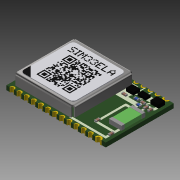
# Autodesk Inventor part: SIM28M
Saved by Autodesk Inventor 2015 SP1 (Build 190203100, 203)
## iProperties
Created: 2015-01-28
Part Number: SIM28M
Material: Типовые
Document SubType Name: Modeling
Designer: Danil
Density: 1 g/cm^3
Appearance: Default
Author: Danil
Autodesk Inventor part; units mm, degrees
(part 1 of 3)
ref_plane "YZ Plane" through (0, 0, 0) normal (1, 0, 0) x (0, 1, 0)
ref_plane "XZ Plane" through (0, 0, 0) normal (0, 1, 0) x (-1, 0, 0)
ref_plane "XY Plane" through (0, 0, 0) normal (0, 0, 1) x (1, 0, 0)
sketch "Эскиз4" plane through (0, 0, 0) normal (0, 0, 1) x (1, 0, 0)
  arc A0 (4.53, 4.775) -> (5.07, 4.775) centre (4.8, 4.775) ccw
  line L0 (5.07, 4.775) -> (5.1, 4.775)
  line L1 (5.1, 4.775) -> (5.1, 4.375) construction
  line L2 (5.1, 4.375) -> (4.5, 4.375) construction
  line L3 (4.5, 4.375) -> (4.5, 4.775) construction
  line L4 (4.5, 4.775) -> (4.53, 4.775)
  arc A1 (4.5, 4.675) -> (5.1, 4.675) centre (4.8, 4.675) ccw
  line L5 (4.8, 4.675) -> (5.1, 4.675) construction
  line L6 (4.8, 4.675) -> (4.5, 4.675) construction
  line L7 (4.5, 4.675) -> (4.5, 4.775)
  line L8 (5.1, 4.775) -> (5.1, 4.675)
  arc A2 (5.68, 4.775) -> (6.22, 4.775) centre (5.95, 4.775) ccw
  arc A3 (5.5, 4.775) -> (6.4, 4.775) centre (5.95, 4.775) ccw
  line L9 (5.5, 4.775) -> (5.68, 4.775)
  line L10 (6.22, 4.775) -> (6.4, 4.775)
  line L11 (-6.975, -4.775) -> (6.975, -4.775)
  line L12 (6.975, -4.775) -> (6.975, 4.775)
  line L13 (6.975, 4.775) -> (-6.975, 4.775)
  line L14 (-6.975, 4.775) -> (-6.975, -4.775)
  line L15 (-6.975, -4.775) -> (6.975, 4.775) construction
  line L16 (6.975, -4.775) -> (-6.975, 4.775) construction
  line L17 (4.53, 4.775) -> (5.07, 4.775)
  line L18 (5.68, 4.775) -> (6.22, 4.775)
  line L19 (0, 0) -> (6.975, 0) construction
  arc A4 (3.53, 4.775) -> (4.07, 4.775) centre (3.8, 4.775) ccw
  line L20 (4.07, 4.775) -> (4.1, 4.775)
  line L21 (4.1, 4.775) -> (4.1, 4.375) construction
  line L22 (4.1, 4.375) -> (3.5, 4.375) construction
  line L23 (3.5, 4.375) -> (3.5, 4.775) construction
  line L24 (3.5, 4.775) -> (3.53, 4.775)
  arc A5 (3.5, 4.675) -> (4.1, 4.675) centre (3.8, 4.675) ccw
  line L25 (3.8, 4.675) -> (4.1, 4.675) construction
  line L26 (3.8, 4.675) -> (3.5, 4.675) construction
  line L27 (3.5, 4.675) -> (3.5, 4.775)
  line L28 (4.1, 4.775) -> (4.1, 4.675)
  line L29 (3.53, 4.775) -> (4.07, 4.775)
  line L30 (2.5, 4.775) -> (2.53, 4.775)
  line L31 (2.8, 4.675) -> (2.5, 4.675) construction
  line L32 (2.53, 4.775) -> (3.07, 4.775)
  arc A6 (2.53, 4.775) -> (3.07, 4.775) centre (2.8, 4.775) ccw
  line L33 (3.07, 4.775) -> (3.1, 4.775)
  line L34 (3.1, 4.775) -> (3.1, 4.375) construction
  line L35 (3.1, 4.375) -> (2.5, 4.375) construction
  line L36 (2.8, 4.675) -> (3.1, 4.675) construction
  arc A7 (2.5, 4.675) -> (3.1, 4.675) centre (2.8, 4.675) ccw
  line L37 (2.5, 4.375) -> (2.5, 4.775) construction
  line L38 (2.5, 4.675) -> (2.5, 4.775)
  line L39 (3.1, 4.775) -> (3.1, 4.675)
  line L40 (1.5, 4.775) -> (1.53, 4.775)
  line L41 (1.8, 4.675) -> (1.5, 4.675) construction
  line L42 (1.53, 4.775) -> (2.07, 4.775)
  arc A8 (1.53, 4.775) -> (2.07, 4.775) centre (1.8, 4.775) ccw
  line L43 (2.07, 4.775) -> (2.1, 4.775)
  line L44 (2.1, 4.775) -> (2.1, 4.375) construction
  line L45 (2.1, 4.375) -> (1.5, 4.375) construction
  line L46 (1.8, 4.675) -> (2.1, 4.675) construction
  arc A9 (1.5, 4.675) -> (2.1, 4.675) centre (1.8, 4.675) ccw
  line L47 (1.5, 4.375) -> (1.5, 4.775) construction
  line L48 (1.5, 4.675) -> (1.5, 4.775)
  line L49 (2.1, 4.775) -> (2.1, 4.675)
  line L50 (0.5, 4.775) -> (0.53, 4.775)
  line L51 (0.8, 4.675) -> (0.5, 4.675) construction
  line L52 (0.53, 4.775) -> (1.07, 4.775)
  arc A10 (0.53, 4.775) -> (1.07, 4.775) centre (0.8, 4.775) ccw
  line L53 (1.07, 4.775) -> (1.1, 4.775)
  line L54 (1.1, 4.775) -> (1.1, 4.375) construction
  line L55 (1.1, 4.375) -> (0.5, 4.375) construction
  line L56 (0.8, 4.675) -> (1.1, 4.675) construction
  arc A11 (0.5, 4.675) -> (1.1, 4.675) centre (0.8, 4.675) ccw
  line L57 (0.5, 4.375) -> (0.5, 4.775) construction
  line L58 (0.5, 4.675) -> (0.5, 4.775)
  line L59 (1.1, 4.775) -> (1.1, 4.675)
  line L60 (-0.5, 4.775) -> (-0.47, 4.775)
  line L61 (-0.2, 4.675) -> (-0.5, 4.675) construction
  line L62 (-0.47, 4.775) -> (0.07, 4.775)
  arc A12 (-0.47, 4.775) -> (0.07, 4.775) centre (-0.2, 4.775) ccw
  line L63 (0.07, 4.775) -> (0.1, 4.775)
  line L64 (0.1, 4.775) -> (0.1, 4.375) construction
  line L65 (0.1, 4.375) -> (-0.5, 4.375) construction
  line L66 (-0.2, 4.675) -> (0.1, 4.675) construction
  arc A13 (-0.5, 4.675) -> (0.1, 4.675) centre (-0.2, 4.675) ccw
  line L67 (-0.5, 4.375) -> (-0.5, 4.775) construction
  line L68 (-0.5, 4.675) -> (-0.5, 4.775)
  line L69 (0.1, 4.775) -> (0.1, 4.675)
  line L70 (-1.5, 4.775) -> (-1.47, 4.775)
  line L71 (-1.2, 4.675) -> (-1.5, 4.675) construction
  line L72 (-1.47, 4.775) -> (-0.93, 4.775)
  arc A14 (-1.47, 4.775) -> (-0.93, 4.775) centre (-1.2, 4.775) ccw
  line L73 (-0.93, 4.775) -> (-0.9, 4.775)
  line L74 (-0.9, 4.775) -> (-0.9, 4.375) construction
  line L75 (-0.9, 4.375) -> (-1.5, 4.375) construction
  line L76 (-1.2, 4.675) -> (-0.9, 4.675) construction
  arc A15 (-1.5, 4.675) -> (-0.9, 4.675) centre (-1.2, 4.675) ccw
  line L77 (-1.5, 4.375) -> (-1.5, 4.775) construction
  line L78 (-1.5, 4.675) -> (-1.5, 4.775)
  line L79 (-0.9, 4.775) -> (-0.9, 4.675)
  line L80 (-2.5, 4.775) -> (-2.47, 4.775)
  line L81 (-2.2, 4.675) -> (-2.5, 4.675) construction
  line L82 (-2.47, 4.775) -> (-1.93, 4.775)
  arc A16 (-2.47, 4.775) -> (-1.93, 4.775) centre (-2.2, 4.775) ccw
  line L83 (-1.93, 4.775) -> (-1.9, 4.775)
  line L84 (-1.9, 4.775) -> (-1.9, 4.375) construction
  line L85 (-1.9, 4.375) -> (-2.5, 4.375) construction
  line L86 (-2.2, 4.675) -> (-1.9, 4.675) construction
  arc A17 (-2.5, 4.675) -> (-1.9, 4.675) centre (-2.2, 4.675) ccw
  line L87 (-2.5, 4.375) -> (-2.5, 4.775) construction
  line L88 (-2.5, 4.675) -> (-2.5, 4.775)
  line L89 (-1.9, 4.775) -> (-1.9, 4.675)
  line L90 (-3.5, 4.775) -> (-3.47, 4.775)
  line L91 (-3.2, 4.675) -> (-3.5, 4.675) construction
  line L92 (-3.47, 4.775) -> (-2.93, 4.775)
  arc A18 (-3.47, 4.775) -> (-2.93, 4.775) centre (-3.2, 4.775) ccw
  line L93 (-2.93, 4.775) -> (-2.9, 4.775)
  line L94 (-2.9, 4.775) -> (-2.9, 4.375) construction
  line L95 (-2.9, 4.375) -> (-3.5, 4.375) construction
  line L96 (-3.2, 4.675) -> (-2.9, 4.675) construction
  arc A19 (-3.5, 4.675) -> (-2.9, 4.675) centre (-3.2, 4.675) ccw
  line L97 (-3.5, 4.375) -> (-3.5, 4.775) construction
  line L98 (-3.5, 4.675) -> (-3.5, 4.775)
  line L99 (-2.9, 4.775) -> (-2.9, 4.675)
  line L100 (-4.5, 4.775) -> (-4.47, 4.775)
  line L101 (-4.2, 4.675) -> (-4.5, 4.675) construction
  line L102 (-4.47, 4.775) -> (-3.93, 4.775)
  arc A20 (-4.47, 4.775) -> (-3.93, 4.775) centre (-4.2, 4.775) ccw
  line L103 (-3.93, 4.775) -> (-3.9, 4.775)
  line L104 (-3.9, 4.775) -> (-3.9, 4.375) construction
  line L105 (-3.9, 4.375) -> (-4.5, 4.375) construction
  line L106 (-4.2, 4.675) -> (-3.9, 4.675) construction
  arc A21 (-4.5, 4.675) -> (-3.9, 4.675) centre (-4.2, 4.675) ccw
  line L107 (-4.5, 4.375) -> (-4.5, 4.775) construction
  line L108 (-4.5, 4.675) -> (-4.5, 4.775)
  line L109 (-3.9, 4.775) -> (-3.9, 4.675)
  line L110 (-5.5, 4.775) -> (-5.47, 4.775)
  line L111 (-5.2, 4.675) -> (-5.5, 4.675) construction
  line L112 (-5.47, 4.775) -> (-4.93, 4.775)
  arc A22 (-5.47, 4.775) -> (-4.93, 4.775) centre (-5.2, 4.775) ccw
  line L113 (-4.93, 4.775) -> (-4.9, 4.775)
  line L114 (-4.9, 4.775) -> (-4.9, 4.375) construction
  line L115 (-4.9, 4.375) -> (-5.5, 4.375) construction
  line L116 (-5.2, 4.675) -> (-4.9, 4.675) construction
  arc A23 (-5.5, 4.675) -> (-4.9, 4.675) centre (-5.2, 4.675) ccw
  line L117 (-5.5, 4.375) -> (-5.5, 4.775) construction
  line L118 (-5.5, 4.675) -> (-5.5, 4.775)
  line L119 (-4.9, 4.775) -> (-4.9, 4.675)
  line L120 (-6.5, 4.775) -> (-6.47, 4.775)
  line L121 (-6.2, 4.675) -> (-6.5, 4.675) construction
  line L122 (-6.47, 4.775) -> (-5.93, 4.775)
  arc A24 (-6.47, 4.775) -> (-5.93, 4.775) centre (-6.2, 4.775) ccw
  line L123 (-5.93, 4.775) -> (-5.9, 4.775)
  line L124 (-5.9, 4.775) -> (-5.9, 4.375) construction
  line L125 (-5.9, 4.375) -> (-6.5, 4.375) construction
  line L126 (-6.2, 4.675) -> (-5.9, 4.675) construction
  arc A25 (-6.5, 4.675) -> (-5.9, 4.675) centre (-6.2, 4.675) ccw
  line L127 (-6.5, 4.375) -> (-6.5, 4.775) construction
  line L128 (-6.5, 4.675) -> (-6.5, 4.775)
  line L129 (-5.9, 4.775) -> (-5.9, 4.675)
  line L130 (-6.875, 1.7) -> (-6.975, 1.7)
  line L131 (-6.575, 1.7) -> (-6.975, 1.7) construction
  line L132 (-6.975, 1.7) -> (-6.975, 1.73)
  line L133 (-6.975, 2.27) -> (-6.975, 2.3)
  arc A26 (-6.875, 1.7) -> (-6.875, 2.3) centre (-6.875, 2) ccw
  line L134 (-6.875, 2) -> (-6.875, 2.3) construction
  line L135 (-6.975, 2.3) -> (-6.875, 2.3)
  line L136 (-6.975, 2.3) -> (-6.575, 2.3) construction
  line L137 (-6.875, 2) -> (-6.875, 1.7) construction
  line L138 (-6.975, 1.73) -> (-6.975, 2.27)
  arc A27 (-6.975, 1.73) -> (-6.975, 2.27) centre (-6.975, 2) ccw
  line L139 (-6.575, 2.3) -> (-6.575, 1.7) construction
  line L140 (-6.975, 1.27) -> (-6.975, 1.3)
  line L141 (-6.875, 1) -> (-6.875, 1.3) construction
  line L142 (-6.975, 1.3) -> (-6.875, 1.3)
  line L143 (-6.975, 1.3) -> (-6.575, 1.3) construction
  line L144 (-6.975, 0.73) -> (-6.975, 1.27)
  arc A28 (-6.975, 0.73) -> (-6.975, 1.27) centre (-6.975, 1) ccw
  line L145 (-6.575, 1.3) -> (-6.575, 0.7) construction
  arc A29 (-6.875, 0.7) -> (-6.875, 1.3) centre (-6.875, 1) ccw
  line L146 (-6.875, 1) -> (-6.875, 0.7) construction
  line L147 (-6.975, 0.7) -> (-6.975, 0.73)
  line L148 (-6.875, 0.7) -> (-6.975, 0.7)
  line L149 (-6.575, 0.7) -> (-6.975, 0.7) construction
  line L150 (-6.975, 0.27) -> (-6.975, 0.3)
  line L151 (-6.875, 0) -> (-6.875, 0.3) construction
  line L152 (-6.975, 0.3) -> (-6.875, 0.3)
  line L153 (-6.975, 0.3) -> (-6.575, 0.3) construction
  line L154 (-6.975, -0.27) -> (-6.975, 0.27)
  arc A30 (-6.975, -0.27) -> (-6.975, 0.27) centre (-6.975, 0) ccw
  line L155 (-6.575, 0.3) -> (-6.575, -0.3) construction
  arc A31 (-6.875, -0.3) -> (-6.875, 0.3) centre (-6.875, 0) ccw
  line L156 (-6.875, 0) -> (-6.875, -0.3) construction
  line L157 (-6.975, -0.3) -> (-6.975, -0.27)
  line L158 (-6.875, -0.3) -> (-6.975, -0.3)
  line L159 (-6.575, -0.3) -> (-6.975, -0.3) construction
  line L160 (-6.975, -0.73) -> (-6.975, -0.7)
  line L161 (-6.875, -1) -> (-6.875, -0.7) construction
  line L162 (-6.975, -0.7) -> (-6.875, -0.7)
  line L163 (-6.975, -0.7) -> (-6.575, -0.7) construction
  line L164 (-6.975, -1.27) -> (-6.975, -0.73)
  arc A32 (-6.975, -1.27) -> (-6.975, -0.73) centre (-6.975, -1) ccw
  line L165 (-6.575, -0.7) -> (-6.575, -1.3) construction
  arc A33 (-6.875, -1.3) -> (-6.875, -0.7) centre (-6.875, -1) ccw
  line L166 (-6.875, -1) -> (-6.875, -1.3) construction
  line L167 (-6.975, -1.3) -> (-6.975, -1.27)
  line L168 (-6.875, -1.3) -> (-6.975, -1.3)
  line L169 (-6.575, -1.3) -> (-6.975, -1.3) construction
  line L170 (-6.975, -1.73) -> (-6.975, -1.7)
  line L171 (-6.875, -2) -> (-6.875, -1.7) construction
  line L172 (-6.975, -1.7) -> (-6.875, -1.7)
  line L173 (-6.975, -1.7) -> (-6.575, -1.7) construction
  line L174 (-6.975, -2.27) -> (-6.975, -1.73)
  arc A34 (-6.975, -2.27) -> (-6.975, -1.73) centre (-6.975, -2) ccw
  line L175 (-6.575, -1.7) -> (-6.575, -2.3) construction
  arc A35 (-6.875, -2.3) -> (-6.875, -1.7) centre (-6.875, -2) ccw
  line L176 (-6.875, -2) -> (-6.875, -2.3) construction
  line L177 (-6.975, -2.3) -> (-6.975, -2.27)
  line L178 (-6.875, -2.3) -> (-6.975, -2.3)
  line L179 (-6.575, -2.3) -> (-6.975, -2.3) construction
  arc A36 (5.07, -4.775) -> (4.53, -4.775) centre (4.8, -4.775) ccw
  line L180 (5.07, -4.775) -> (5.1, -4.775)
  line L181 (5.1, -4.775) -> (5.1, -4.375) construction
  line L182 (5.1, -4.375) -> (4.5, -4.375) construction
  line L183 (4.5, -4.375) -> (4.5, -4.775) construction
  line L184 (4.5, -4.775) -> (4.53, -4.775)
  arc A37 (5.1, -4.675) -> (4.5, -4.675) centre (4.8, -4.675) ccw
  line L185 (4.8, -4.675) -> (5.1, -4.675) construction
  line L186 (4.8, -4.675) -> (4.5, -4.675) construction
  line L187 (4.5, -4.675) -> (4.5, -4.775)
  line L188 (5.1, -4.775) -> (5.1, -4.675)
  arc A38 (6.22, -4.775) -> (5.68, -4.775) centre (5.95, -4.775) ccw
  arc A39 (6.4, -4.775) -> (5.5, -4.775) centre (5.95, -4.775) ccw
  line L189 (5.5, -4.775) -> (5.68, -4.775)
  line L190 (6.22, -4.775) -> (6.4, -4.775)
  line L191 (4.53, -4.775) -> (5.07, -4.775)
  line L192 (5.68, -4.775) -> (6.22, -4.775)
  line L193 (3.5, -4.775) -> (3.53, -4.775)
  line L194 (3.8, -4.675) -> (3.5, -4.675) construction
  line L195 (3.53, -4.775) -> (4.07, -4.775)
  arc A40 (4.07, -4.775) -> (3.53, -4.775) centre (3.8, -4.775) ccw
  line L196 (4.07, -4.775) -> (4.1, -4.775)
  line L197 (4.1, -4.775) -> (4.1, -4.375) construction
  line L198 (4.1, -4.375) -> (3.5, -4.375) construction
  line L199 (3.8, -4.675) -> (4.1, -4.675) construction
  arc A41 (4.1, -4.675) -> (3.5, -4.675) centre (3.8, -4.675) ccw
  line L200 (3.5, -4.375) -> (3.5, -4.775) construction
  line L201 (3.5, -4.675) -> (3.5, -4.775)
  line L202 (4.1, -4.775) -> (4.1, -4.675)
  line L203 (2.5, -4.675) -> (2.5, -4.775)
  line L204 (2.5, -4.375) -> (2.5, -4.775) construction
  line L205 (2.5, -4.775) -> (2.53, -4.775)
  line L206 (3.07, -4.775) -> (3.1, -4.775)
  arc A42 (3.1, -4.675) -> (2.5, -4.675) centre (2.8, -4.675) ccw
  line L207 (2.8, -4.675) -> (3.1, -4.675) construction
  line L208 (3.1, -4.775) -> (3.1, -4.675)
  line L209 (3.1, -4.775) -> (3.1, -4.375) construction
  line L210 (2.8, -4.675) -> (2.5, -4.675) construction
  line L211 (2.53, -4.775) -> (3.07, -4.775)
  arc A43 (3.07, -4.775) -> (2.53, -4.775) centre (2.8, -4.775) ccw
  line L212 (3.1, -4.375) -> (2.5, -4.375) construction
  line L213 (1.5, -4.675) -> (1.5, -4.775)
  line L214 (1.5, -4.375) -> (1.5, -4.775) construction
  line L215 (1.5, -4.775) -> (1.53, -4.775)
  line L216 (2.07, -4.775) -> (2.1, -4.775)
  arc A44 (2.1, -4.675) -> (1.5, -4.675) centre (1.8, -4.675) ccw
  line L217 (1.8, -4.675) -> (2.1, -4.675) construction
  line L218 (2.1, -4.775) -> (2.1, -4.675)
  line L219 (2.1, -4.775) -> (2.1, -4.375) construction
  line L220 (1.8, -4.675) -> (1.5, -4.675) construction
  line L221 (1.53, -4.775) -> (2.07, -4.775)
  arc A45 (2.07, -4.775) -> (1.53, -4.775) centre (1.8, -4.775) ccw
  line L222 (2.1, -4.375) -> (1.5, -4.375) construction
  line L223 (0.5, -4.675) -> (0.5, -4.775)
  line L224 (0.5, -4.375) -> (0.5, -4.775) construction
  line L225 (0.5, -4.775) -> (0.53, -4.775)
  line L226 (1.07, -4.775) -> (1.1, -4.775)
  arc A46 (1.1, -4.675) -> (0.5, -4.675) centre (0.8, -4.675) ccw
  line L227 (0.8, -4.675) -> (1.1, -4.675) construction
  line L228 (1.1, -4.775) -> (1.1, -4.675)
  line L229 (1.1, -4.775) -> (1.1, -4.375) construction
  line L230 (0.8, -4.675) -> (0.5, -4.675) construction
  line L231 (0.53, -4.775) -> (1.07, -4.775)
  arc A47 (1.07, -4.775) -> (0.53, -4.775) centre (0.8, -4.775) ccw
  line L232 (1.1, -4.375) -> (0.5, -4.375) construction
  line L233 (-0.5, -4.675) -> (-0.5, -4.775)
  line L234 (-0.5, -4.375) -> (-0.5, -4.775) construction
  line L235 (-0.5, -4.775) -> (-0.47, -4.775)
  line L236 (0.07, -4.775) -> (0.1, -4.775)
  arc A48 (0.1, -4.675) -> (-0.5, -4.675) centre (-0.2, -4.675) ccw
  line L237 (-0.2, -4.675) -> (0.1, -4.675) construction
  line L238 (0.1, -4.775) -> (0.1, -4.675)
  line L239 (0.1, -4.775) -> (0.1, -4.375) construction
  line L240 (-0.2, -4.675) -> (-0.5, -4.675) construction
  line L241 (-0.47, -4.775) -> (0.07, -4.775)
  arc A49 (0.07, -4.775) -> (-0.47, -4.775) centre (-0.2, -4.775) ccw
  line L242 (0.1, -4.375) -> (-0.5, -4.375) construction
  line L243 (-1.5, -4.675) -> (-1.5, -4.775)
  line L244 (-1.5, -4.375) -> (-1.5, -4.775) construction
  line L245 (-1.5, -4.775) -> (-1.47, -4.775)
  line L246 (-0.93, -4.775) -> (-0.9, -4.775)
  arc A50 (-0.9, -4.675) -> (-1.5, -4.675) centre (-1.2, -4.675) ccw
  line L247 (-1.2, -4.675) -> (-0.9, -4.675) construction
  line L248 (-0.9, -4.775) -> (-0.9, -4.675)
  line L249 (-0.9, -4.775) -> (-0.9, -4.375) construction
  line L250 (-1.2, -4.675) -> (-1.5, -4.675) construction
  line L251 (-1.47, -4.775) -> (-0.93, -4.775)
  arc A51 (-0.93, -4.775) -> (-1.47, -4.775) centre (-1.2, -4.775) ccw
  line L252 (-0.9, -4.375) -> (-1.5, -4.375) construction
  line L253 (-2.5, -4.675) -> (-2.5, -4.775)
  line L254 (-2.5, -4.375) -> (-2.5, -4.775) construction
  line L255 (-2.5, -4.775) -> (-2.47, -4.775)
  line L256 (-1.93, -4.775) -> (-1.9, -4.775)
  arc A52 (-1.9, -4.675) -> (-2.5, -4.675) centre (-2.2, -4.675) ccw
  line L257 (-2.2, -4.675) -> (-1.9, -4.675) construction
  line L258 (-1.9, -4.775) -> (-1.9, -4.675)
  line L259 (-1.9, -4.775) -> (-1.9, -4.375) construction
  line L260 (-2.2, -4.675) -> (-2.5, -4.675) construction
  line L261 (-2.47, -4.775) -> (-1.93, -4.775)
  arc A53 (-1.93, -4.775) -> (-2.47, -4.775) centre (-2.2, -4.775) ccw
  line L262 (-1.9, -4.375) -> (-2.5, -4.375) construction
  line L263 (-3.5, -4.675) -> (-3.5, -4.775)
  line L264 (-3.5, -4.375) -> (-3.5, -4.775) construction
  line L265 (-3.5, -4.775) -> (-3.47, -4.775)
  line L266 (-2.93, -4.775) -> (-2.9, -4.775)
  arc A54 (-2.9, -4.675) -> (-3.5, -4.675) centre (-3.2, -4.675) ccw
  line L267 (-3.2, -4.675) -> (-2.9, -4.675) construction
  line L268 (-2.9, -4.775) -> (-2.9, -4.675)
  line L269 (-2.9, -4.775) -> (-2.9, -4.375) construction
  line L270 (-3.2, -4.675) -> (-3.5, -4.675) construction
  line L271 (-3.47, -4.775) -> (-2.93, -4.775)
  arc A55 (-2.93, -4.775) -> (-3.47, -4.775) centre (-3.2, -4.775) ccw
  line L272 (-2.9, -4.375) -> (-3.5, -4.375) construction
  line L273 (-4.5, -4.675) -> (-4.5, -4.775)
  line L274 (-4.5, -4.375) -> (-4.5, -4.775) construction
  line L275 (-4.5, -4.775) -> (-4.47, -4.775)
  line L276 (-3.93, -4.775) -> (-3.9, -4.775)
  arc A56 (-3.9, -4.675) -> (-4.5, -4.675) centre (-4.2, -4.675) ccw
  line L277 (-4.2, -4.675) -> (-3.9, -4.675) construction
  line L278 (-3.9, -4.775) -> (-3.9, -4.675)
  line L279 (-3.9, -4.775) -> (-3.9, -4.375) construction
  line L280 (-4.2, -4.675) -> (-4.5, -4.675) construction
  line L281 (-4.47, -4.775) -> (-3.93, -4.775)
  arc A57 (-3.93, -4.775) -> (-4.47, -4.775) centre (-4.2, -4.775) ccw
  line L282 (-3.9, -4.375) -> (-4.5, -4.375) construction
  line L283 (-5.5, -4.675) -> (-5.5, -4.775)
  line L284 (-5.5, -4.375) -> (-5.5, -4.775) construction
  line L285 (-5.5, -4.775) -> (-5.47, -4.775)
  line L286 (-4.93, -4.775) -> (-4.9, -4.775)
  arc A58 (-4.9, -4.675) -> (-5.5, -4.675) centre (-5.2, -4.675) ccw
  line L287 (-5.2, -4.675) -> (-4.9, -4.675) construction
  line L288 (-4.9, -4.775) -> (-4.9, -4.675)
  line L289 (-4.9, -4.775) -> (-4.9, -4.375) construction
  line L290 (-5.2, -4.675) -> (-5.5, -4.675) construction
  line L291 (-5.47, -4.775) -> (-4.93, -4.775)
  arc A59 (-4.93, -4.775) -> (-5.47, -4.775) centre (-5.2, -4.775) ccw
  line L292 (-4.9, -4.375) -> (-5.5, -4.375) construction
  line L293 (-6.5, -4.675) -> (-6.5, -4.775)
  line L294 (-6.5, -4.375) -> (-6.5, -4.775) construction
  line L295 (-6.5, -4.775) -> (-6.47, -4.775)
  line L296 (-5.93, -4.775) -> (-5.9, -4.775)
  arc A60 (-5.9, -4.675) -> (-6.5, -4.675) centre (-6.2, -4.675) ccw
  line L297 (-6.2, -4.675) -> (-5.9, -4.675) construction
  line L298 (-5.9, -4.775) -> (-5.9, -4.675)
  line L299 (-5.9, -4.775) -> (-5.9, -4.375) construction
  line L300 (-6.2, -4.675) -> (-6.5, -4.675) construction
  line L301 (-6.47, -4.775) -> (-5.93, -4.775)
  arc A61 (-5.93, -4.775) -> (-6.47, -4.775) centre (-6.2, -4.775) ccw
  line L302 (-5.9, -4.375) -> (-6.5, -4.375) construction
  point P0 (4.8, 4.375)
  point P1 (3.8, 4.375)
  point P2 (2.8, 4.375)
  point P3 (1.8, 4.375)
  point P4 (0.8, 4.375)
  point P5 (-0.2, 4.375)
  point P6 (-1.2, 4.375)
  point P7 (-2.2, 4.375)
  point P8 (-3.2, 4.375)
  point P9 (-4.2, 4.375)
  point P10 (-5.2, 4.375)
  point P11 (-6.2, 4.375)
  point P12 (-6.575, 2)
  point P13 (-6.575, 1)
  point P14 (-6.575, 0)
  point P15 (-6.575, -1)
  point P16 (-6.575, -2)
  point P17 (-6.975, 0)
  point P18 (4.8, -4.375)
  point P19 (3.8, -4.375)
  point P20 (2.8, -4.375)
  point P21 (1.8, -4.375)
  point P22 (0.8, -4.375)
  point P23 (-0.2, -4.375)
  point P24 (-1.2, -4.375)
  point P25 (-2.2, -4.375)
  point P26 (-3.2, -4.375)
  point P27 (-4.2, -4.375)
  point P28 (-5.2, -4.375)
  point P29 (-6.2, -4.375)
  dimension "d738" = 0.27
  dimension "d741" = 0.6
  dimension "d742" = 0.4
  dimension "d809" = 0.27
  dimension "d826" = 0.45
  dimension "d830" = 1.15
  dimension "d872" = 13.95
  dimension "d873" = 9.55
  dimension "d874" = 0.27
  dimension "d875" = 0.6
  dimension "d876" = 0.4
  dimension "d877" = 1
  dimension "d878" = 0.27
  dimension "d879" = 0.6
  dimension "d880" = 0.4
  dimension "d881" = 0.27
  dimension "d882" = 0.6
  dimension "d883" = 0.4
  dimension "d884" = 0.27
  dimension "d885" = 0.6
  dimension "d886" = 0.4
  dimension "d887" = 0.27
  dimension "d888" = 0.6
  dimension "d889" = 0.4
  dimension "d890" = 0.27
  dimension "d891" = 0.6
  dimension "d892" = 0.4
  dimension "d893" = 0.27
  dimension "d894" = 0.6
  dimension "d895" = 0.4
  dimension "d896" = 0.27
  dimension "d897" = 0.6
  dimension "d898" = 0.4
  dimension "d899" = 0.27
  dimension "d900" = 0.6
  dimension "d901" = 0.4
  dimension "d902" = 0.27
  dimension "d903" = 0.6
  dimension "d904" = 0.4
  dimension "d905" = 0.27
  dimension "d906" = 0.6
  dimension "d907" = 0.4
  dimension "d908" = 1
  dimension "d909" = 0.775
  dimension "d910" = 1
  dimension "d911" = 1
  dimension "d912" = 1
  dimension "d913" = 1
  dimension "d914" = 1
  dimension "d915" = 1
  dimension "d916" = 1
  dimension "d917" = 1
  dimension "d918" = 1
  dimension "d919" = 0.27
  dimension "d920" = 0.6
  dimension "d921" = 0.4
  dimension "d923" = 2.775
  dimension "d924" = 0.27
  dimension "d925" = 0.6
  dimension "d926" = 0.4
  dimension "d927" = 0.27
  dimension "d928" = 0.6
  dimension "d929" = 0.4
  dimension "d930" = 0.27
  constraints: 604 end point, 149 symmetric about line, 141 point on circle, 91 point on line, 86 perpendicular, 62 centre point, 57 horizontal alignment, 39 midpoint, 35 parallel, 18 collinear, 17 horizontal, 17 vertical alignment, 7 coincident, 43 other
  measures "d738" radius of A0
  measures "d741" distance between parallel lines of L1 L3
  measures "d742" distance of L2.end L3.end
  measures "d809" radius of A2
  measures "d826" radius of A3
  measures "d830" distance of A0.centre A2.centre
  measures "d872" distance of L14.start L12.end
  measures "d873" distance of L12.end L11.end
  measures "d874" radius of A4
  measures "d875" distance between parallel lines of L21 L23
  measures "d876" distance of L22.end L24.start
  measures "d877" distance of A0.centre A4.centre
  measures "d878" radius of A6
  measures "d879" distance between parallel lines of L34 L37
  measures "d880" distance of L37.start L38.end
  measures "d881" radius of A8
  measures "d882" distance between parallel lines of L44 L47
  measures "d883" distance of L47.start L48.end
  measures "d884" radius of A10
  measures "d885" distance between parallel lines of L54 L57
  measures "d886" distance of L57.start L58.end
  measures "d887" radius of A12
  measures "d888" distance between parallel lines of L64 L67
  measures "d889" distance of L67.start L68.end
  measures "d890" radius of A14
  measures "d891" distance between parallel lines of L74 L77
  measures "d892" distance of L77.start L78.end
  measures "d893" radius of A16
  measures "d894" distance between parallel lines of L84 L87
  measures "d895" distance of L87.start L88.end
  measures "d896" radius of A18
  measures "d897" distance between parallel lines of L94 L97
  measures "d898" distance of L97.start L98.end
  measures "d899" radius of A20
  measures "d900" distance between parallel lines of L104 L107
  measures "d901" distance of L107.start L108.end
  measures "d902" radius of A22
  measures "d903" distance between parallel lines of L114 L117
  measures "d904" distance of L117.start L118.end
  measures "d905" radius of A24
  measures "d906" distance between parallel lines of L124 L127
  measures "d907" distance of L127.start L128.end
  measures "d908" distance of A4.centre A6.centre
  measures "d909" distance of L14.start A24.centre
  measures "d910" distance of A22.centre A24.centre
  measures "d911" distance of point (-4.2, 4.775) A22.centre
  measures "d912" distance of A18.centre A20.centre
  measures "d913" distance of A16.centre A18.centre
  measures "d914" distance of A14.centre point (-2.2, 4.775)
  measures "d915" distance of A12.centre A14.centre
  measures "d916" distance of A12.centre A10.centre
  measures "d917" distance of A10.centre A8.centre
  measures "d918" distance of A8.centre A6.centre
  measures "d919" radius of A27
  measures "d920" distance between parallel lines of L136 L131
  measures "d921" distance of L139.end L132.start
  measures "d923" distance of L14.start A27.centre
  measures "d924" radius of A28
  measures "d925" distance between parallel lines of L143 L149
  measures "d926" distance of L149.start L147.start
  measures "d927" radius of A30
  measures "d928" distance between parallel lines of L153 L159
  measures "d929" distance of L159.start L157.start
  measures "d930" radius of A32
extrude "Extrusion19" add sketch "Эскиз4" along normal blind 0.6 contours A0 L0 L8 A1 L7 L4 | L7 A1 L8 L13 A3 L12 L11 A39 L188 A37 L187 L202 A41 L201 L208 A42 L203 L218 A44 L213 L228 A46 L223 L238 A48 L233 L248 A50 L243 L258 A52 L253 L268 A54 L263 L278 A56 L273 L288 A58 L283 L298 A60 L293 L14 L178 A35 L172 L168 A33 L162 L158 A31 L152 L148 A29 L142 L130 A26 L135 L128 A25 L129 L118 A23 L119 L108 A21 L109 L98 A19 L99 L88 A17 L89 L78 A15 L79 L68 A13 L69 L58 A11 L59 L48 A9 L49 L38 A7 L39 L27 A5 L28 | L28 A5 L27 L13 A4 | L9 A2 L10 A3 | L39 A7 L38 L13 A6 | L11 A38 A39 | L11 A36 L187 A37 L188 | L49 A9 L48 L13 A8 | L11 A40 L201 A41 L202 | L59 A11 L58 L13 A10 | L11 A43 L203 A42 L208 | L69 A13 L68 L13 A12 | L11 A45 L213 A44 L218 | L79 A15 L78 L13 A14 | L11 A47 L223 A46 L228 | L89 A17 L88 L13 A16 | L11 A49 L233 A48 L238 | L99 A19 L98 L13 A18 | L11 A51 L243 A50 L248 | L109 A21 L108 L13 A20 | L11 A53 L253 A52 L258 | L119 A23 L118 L13 A22 | L11 A55 L263 A54 L268 | L129 A25 L128 L13 A24 | L11 A57 L273 A56 L278 | L135 A26 L130 L14 A27 | L11 A59 L283 A58 L288 | L142 A29 L148 L14 A28 | L11 A61 L293 A60 L298 | L152 A31 L158 L14 A30 | L14 A34 L172 A35 L178 | L162 A33 L168 L14 A32
sketch "Sketch20" plane through (0, 0, 0) normal (0, 0, 1) x (1, 0, 0)
  arc A0 (4.55, 4.8) -> (5.05, 4.8) centre (4.8, 4.8) ccw
  line L0 (5.05, 4.8) -> (5.1, 4.8)
  line L1 (5.1, 4.8) -> (5.1, 4.4) construction
  line L2 (5.1, 4.4) -> (4.5, 4.4) construction
  line L3 (4.5, 4.4) -> (4.5, 4.8) construction
  line L4 (4.5, 4.8) -> (4.55, 4.8)
  arc A1 (4.5, 4.7) -> (5.1, 4.7) centre (4.8, 4.7) ccw
  line L5 (4.8, 4.7) -> (5.1, 4.7) construction
  line L6 (4.8, 4.7) -> (4.5, 4.7) construction
  line L7 (4.5, 4.7) -> (4.5, 4.8)
  line L8 (5.1, 4.8) -> (5.1, 4.7)
  arc A2 (5.7, 4.8) -> (6.2, 4.8) centre (5.95, 4.8) ccw
  arc A3 (5.5, 4.8) -> (6.4, 4.8) centre (5.95, 4.8) ccw
  line L9 (5.5, 4.8) -> (5.7, 4.8)
  line L10 (6.2, 4.8) -> (6.4, 4.8)
  line L11 (-7, -4.8) -> (7, -4.8)
  line L12 (7, -4.8) -> (7, 4.8)
  line L13 (7, 4.8) -> (-7, 4.8)
  line L14 (-7, 4.8) -> (-7, -4.8)
  line L15 (-7, -4.8) -> (7, 4.8) construction
  line L16 (7, -4.8) -> (-7, 4.8) construction
  line L17 (4.55, 4.8) -> (5.05, 4.8)
  line L18 (5.7, 4.8) -> (6.2, 4.8)
  line L19 (0, 0) -> (7, 0) construction
  line L20 (-7, 2.25) -> (-7, 2.3)
  line L21 (-6.9, 2) -> (-6.9, 2.3) construction
  line L22 (-7, 2.3) -> (-6.9, 2.3)
  line L23 (-7, 2.3) -> (-6.6, 2.3) construction
  line L24 (-7, 1.75) -> (-7, 2.25)
  arc A4 (-7, 1.75) -> (-7, 2.25) centre (-7, 2) ccw
  line L25 (-6.6, 2.3) -> (-6.6, 1.7) construction
  arc A5 (-6.9, 1.7) -> (-6.9, 2.3) centre (-6.9, 2) ccw
  line L26 (-6.9, 2) -> (-6.9, 1.7) construction
  line L27 (-7, 1.7) -> (-7, 1.75)
  line L28 (-6.9, 1.7) -> (-7, 1.7)
  line L29 (-6.6, 1.7) -> (-7, 1.7) construction
  line L30 (4.5, 4.8) -> (4.5, 3.8)
  line L31 (4.5, 3.8) -> (5.1, 3.8)
  line L32 (5.1, 3.8) -> (5.1, 4.8)
  arc A6 (3.55, 4.8) -> (4.05, 4.8) centre (3.8, 4.8) ccw
  line L33 (4.05, 4.8) -> (4.1, 4.8)
  line L34 (4.1, 4.8) -> (4.1, 4.4) construction
  line L35 (4.1, 4.4) -> (3.5, 4.4) construction
  line L36 (3.5, 4.4) -> (3.5, 4.8) construction
  line L37 (3.5, 4.8) -> (3.55, 4.8)
  arc A7 (3.5, 4.7) -> (4.1, 4.7) centre (3.8, 4.7) ccw
  line L38 (3.8, 4.7) -> (4.1, 4.7) construction
  line L39 (3.8, 4.7) -> (3.5, 4.7) construction
  line L40 (3.5, 4.7) -> (3.5, 4.8)
  line L41 (4.1, 4.8) -> (4.1, 4.7)
  line L42 (3.55, 4.8) -> (4.05, 4.8)
  line L43 (3.5, 4.8) -> (3.5, 3.8)
  line L44 (3.5, 3.8) -> (4.1, 3.8)
  line L45 (4.1, 3.8) -> (4.1, 4.8)
  arc A8 (2.55, 4.8) -> (3.05, 4.8) centre (2.8, 4.8) ccw
  line L46 (3.05, 4.8) -> (3.1, 4.8)
  line L47 (3.1, 4.8) -> (3.1, 4.4) construction
  line L48 (3.1, 4.4) -> (2.5, 4.4) construction
  line L49 (2.5, 4.4) -> (2.5, 4.8) construction
  line L50 (2.5, 4.8) -> (2.55, 4.8)
  arc A9 (2.5, 4.7) -> (3.1, 4.7) centre (2.8, 4.7) ccw
  line L51 (2.8, 4.7) -> (3.1, 4.7) construction
  line L52 (2.8, 4.7) -> (2.5, 4.7) construction
  line L53 (2.5, 4.7) -> (2.5, 4.8)
  line L54 (3.1, 4.8) -> (3.1, 4.7)
  line L55 (2.55, 4.8) -> (3.05, 4.8)
  line L56 (2.5, 4.8) -> (2.5, 3.8)
  line L57 (2.5, 3.8) -> (3.1, 3.8)
  line L58 (3.1, 3.8) -> (3.1, 4.8)
  arc A10 (1.55, 4.8) -> (2.05, 4.8) centre (1.8, 4.8) ccw
  line L59 (2.05, 4.8) -> (2.1, 4.8)
  line L60 (2.1, 4.8) -> (2.1, 4.4) construction
  line L61 (2.1, 4.4) -> (1.5, 4.4) construction
  line L62 (1.5, 4.4) -> (1.5, 4.8) construction
  line L63 (1.5, 4.8) -> (1.55, 4.8)
  arc A11 (1.5, 4.7) -> (2.1, 4.7) centre (1.8, 4.7) ccw
  line L64 (1.8, 4.7) -> (2.1, 4.7) construction
  line L65 (1.8, 4.7) -> (1.5, 4.7) construction
  line L66 (1.5, 4.7) -> (1.5, 4.8)
  line L67 (2.1, 4.8) -> (2.1, 4.7)
  line L68 (1.55, 4.8) -> (2.05, 4.8)
  line L69 (1.5, 4.8) -> (1.5, 3.8)
  line L70 (1.5, 3.8) -> (2.1, 3.8)
  line L71 (2.1, 3.8) -> (2.1, 4.8)
  arc A12 (0.55, 4.8) -> (1.05, 4.8) centre (0.8, 4.8) ccw
  line L72 (1.05, 4.8) -> (1.1, 4.8)
  line L73 (1.1, 4.8) -> (1.1, 4.4) construction
  line L74 (1.1, 4.4) -> (0.5, 4.4) construction
  line L75 (0.5, 4.4) -> (0.5, 4.8) construction
  line L76 (0.5, 4.8) -> (0.55, 4.8)
  arc A13 (0.5, 4.7) -> (1.1, 4.7) centre (0.8, 4.7) ccw
  line L77 (0.8, 4.7) -> (1.1, 4.7) construction
  line L78 (0.8, 4.7) -> (0.5, 4.7) construction
  line L79 (0.5, 4.7) -> (0.5, 4.8)
  line L80 (1.1, 4.8) -> (1.1, 4.7)
  line L81 (0.55, 4.8) -> (1.05, 4.8)
  line L82 (0.5, 4.8) -> (0.5, 3.8)
  line L83 (0.5, 3.8) -> (1.1, 3.8)
  line L84 (1.1, 3.8) -> (1.1, 4.8)
  arc A14 (-0.45, 4.8) -> (0.05, 4.8) centre (-0.2, 4.8) ccw
  line L85 (0.05, 4.8) -> (0.1, 4.8)
  line L86 (0.1, 4.8) -> (0.1, 4.4) construction
  line L87 (0.1, 4.4) -> (-0.5, 4.4) construction
  line L88 (-0.5, 4.4) -> (-0.5, 4.8) construction
  line L89 (-0.5, 4.8) -> (-0.45, 4.8)
  arc A15 (-0.5, 4.7) -> (0.1, 4.7) centre (-0.2, 4.7) ccw
  line L90 (-0.2, 4.7) -> (0.1, 4.7) construction
  line L91 (-0.2, 4.7) -> (-0.5, 4.7) construction
  line L92 (-0.5, 4.7) -> (-0.5, 4.8)
  line L93 (0.1, 4.8) -> (0.1, 4.7)
  line L94 (-0.45, 4.8) -> (0.05, 4.8)
  line L95 (-0.5, 4.8) -> (-0.5, 3.8)
  line L96 (-0.5, 3.8) -> (0.1, 3.8)
  line L97 (0.1, 3.8) -> (0.1, 4.8)
  arc A16 (-1.45, 4.8) -> (-0.95, 4.8) centre (-1.2, 4.8) ccw
  line L98 (-0.95, 4.8) -> (-0.9, 4.8)
  line L99 (-0.9, 4.8) -> (-0.9, 4.4) construction
  line L100 (-0.9, 4.4) -> (-1.5, 4.4) construction
  line L101 (-1.5, 4.4) -> (-1.5, 4.8) construction
  line L102 (-1.5, 4.8) -> (-1.45, 4.8)
  arc A17 (-1.5, 4.7) -> (-0.9, 4.7) centre (-1.2, 4.7) ccw
  line L103 (-1.2, 4.7) -> (-0.9, 4.7) construction
  line L104 (-1.2, 4.7) -> (-1.5, 4.7) construction
  line L105 (-1.5, 4.7) -> (-1.5, 4.8)
  line L106 (-0.9, 4.8) -> (-0.9, 4.7)
  line L107 (-1.45, 4.8) -> (-0.95, 4.8)
  line L108 (-1.5, 4.8) -> (-1.5, 3.8)
  line L109 (-1.5, 3.8) -> (-0.9, 3.8)
  line L110 (-0.9, 3.8) -> (-0.9, 4.8)
  arc A18 (-2.45, 4.8) -> (-1.95, 4.8) centre (-2.2, 4.8) ccw
  line L111 (-1.95, 4.8) -> (-1.9, 4.8)
  line L112 (-1.9, 4.8) -> (-1.9, 4.4) construction
  line L113 (-1.9, 4.4) -> (-2.5, 4.4) construction
  line L114 (-2.5, 4.4) -> (-2.5, 4.8) construction
  line L115 (-2.5, 4.8) -> (-2.45, 4.8)
  arc A19 (-2.5, 4.7) -> (-1.9, 4.7) centre (-2.2, 4.7) ccw
  line L116 (-2.2, 4.7) -> (-1.9, 4.7) construction
  line L117 (-2.2, 4.7) -> (-2.5, 4.7) construction
  line L118 (-2.5, 4.7) -> (-2.5, 4.8)
  line L119 (-1.9, 4.8) -> (-1.9, 4.7)
  line L120 (-2.45, 4.8) -> (-1.95, 4.8)
  line L121 (-2.5, 4.8) -> (-2.5, 3.8)
  line L122 (-2.5, 3.8) -> (-1.9, 3.8)
  line L123 (-1.9, 3.8) -> (-1.9, 4.8)
  arc A20 (-3.45, 4.8) -> (-2.95, 4.8) centre (-3.2, 4.8) ccw
  line L124 (-2.95, 4.8) -> (-2.9, 4.8)
  line L125 (-2.9, 4.8) -> (-2.9, 4.4) construction
  line L126 (-2.9, 4.4) -> (-3.5, 4.4) construction
  line L127 (-3.5, 4.4) -> (-3.5, 4.8) construction
  line L128 (-3.5, 4.8) -> (-3.45, 4.8)
  arc A21 (-3.5, 4.7) -> (-2.9, 4.7) centre (-3.2, 4.7) ccw
  line L129 (-3.2, 4.7) -> (-2.9, 4.7) construction
  line L130 (-3.2, 4.7) -> (-3.5, 4.7) construction
  line L131 (-3.5, 4.7) -> (-3.5, 4.8)
  line L132 (-2.9, 4.8) -> (-2.9, 4.7)
  line L133 (-3.45, 4.8) -> (-2.95, 4.8)
  line L134 (-3.5, 4.8) -> (-3.5, 3.8)
  line L135 (-3.5, 3.8) -> (-2.9, 3.8)
  line L136 (-2.9, 3.8) -> (-2.9, 4.8)
  arc A22 (-4.45, 4.8) -> (-3.95, 4.8) centre (-4.2, 4.8) ccw
  line L137 (-3.95, 4.8) -> (-3.9, 4.8)
  line L138 (-3.9, 4.8) -> (-3.9, 4.4) construction
  line L139 (-3.9, 4.4) -> (-4.5, 4.4) construction
  line L140 (-4.5, 4.4) -> (-4.5, 4.8) construction
  line L141 (-4.5, 4.8) -> (-4.45, 4.8)
  arc A23 (-4.5, 4.7) -> (-3.9, 4.7) centre (-4.2, 4.7) ccw
  line L142 (-4.2, 4.7) -> (-3.9, 4.7) construction
  line L143 (-4.2, 4.7) -> (-4.5, 4.7) construction
  line L144 (-4.5, 4.7) -> (-4.5, 4.8)
  line L145 (-3.9, 4.8) -> (-3.9, 4.7)
  line L146 (-4.45, 4.8) -> (-3.95, 4.8)
  line L147 (-4.5, 4.8) -> (-4.5, 3.8)
  line L148 (-4.5, 3.8) -> (-3.9, 3.8)
  line L149 (-3.9, 3.8) -> (-3.9, 4.8)
  arc A24 (-5.45, 4.8) -> (-4.95, 4.8) centre (-5.2, 4.8) ccw
  line L150 (-4.95, 4.8) -> (-4.9, 4.8)
  line L151 (-4.9, 4.8) -> (-4.9, 4.4) construction
  line L152 (-4.9, 4.4) -> (-5.5, 4.4) construction
  line L153 (-5.5, 4.4) -> (-5.5, 4.8) construction
  line L154 (-5.5, 4.8) -> (-5.45, 4.8)
  arc A25 (-5.5, 4.7) -> (-4.9, 4.7) centre (-5.2, 4.7) ccw
  line L155 (-5.2, 4.7) -> (-4.9, 4.7) construction
  line L156 (-5.2, 4.7) -> (-5.5, 4.7) construction
  line L157 (-5.5, 4.7) -> (-5.5, 4.8)
  line L158 (-4.9, 4.8) -> (-4.9, 4.7)
  line L159 (-5.45, 4.8) -> (-4.95, 4.8)
  line L160 (-5.5, 4.8) -> (-5.5, 3.8)
  line L161 (-5.5, 3.8) -> (-4.9, 3.8)
  line L162 (-4.9, 3.8) -> (-4.9, 4.8)
  arc A26 (-6.45, 4.8) -> (-5.95, 4.8) centre (-6.2, 4.8) ccw
  line L163 (-5.95, 4.8) -> (-5.9, 4.8)
  line L164 (-5.9, 4.8) -> (-5.9, 4.4) construction
  line L165 (-5.9, 4.4) -> (-6.5, 4.4) construction
  line L166 (-6.5, 4.4) -> (-6.5, 4.8) construction
  line L167 (-6.5, 4.8) -> (-6.45, 4.8)
  arc A27 (-6.5, 4.7) -> (-5.9, 4.7) centre (-6.2, 4.7) ccw
  line L168 (-6.2, 4.7) -> (-5.9, 4.7) construction
  line L169 (-6.2, 4.7) -> (-6.5, 4.7) construction
  line L170 (-6.5, 4.7) -> (-6.5, 4.8)
  line L171 (-5.9, 4.8) -> (-5.9, 4.7)
  line L172 (-6.45, 4.8) -> (-5.95, 4.8)
  line L173 (-6.5, 4.8) -> (-6.5, 3.8)
  line L174 (-6.5, 3.8) -> (-5.9, 3.8)
  line L175 (-5.9, 3.8) -> (-5.9, 4.8)
  line L176 (5.5, 4.8) -> (6.4, 4.8)
  line L177 (6.4, 4.8) -> (6.4, 3.8)
  line L178 (6.4, 3.8) -> (5.5, 3.8)
  line L179 (5.5, 3.8) -> (5.5, 4.8)
  line L180 (-7, 1.7) -> (-6, 1.7)
  line L181 (-6, 1.7) -> (-6, 2.3)
  line L182 (-6, 2.3) -> (-7, 2.3)
  line L183 (-7, 2.3) -> (-7, 1.7)
  line L184 (-7, 1.25) -> (-7, 1.3)
  line L185 (-6.9, 1) -> (-6.9, 1.3) construction
  line L186 (-7, 1.3) -> (-6.9, 1.3)
  line L187 (-7, 1.3) -> (-6.6, 1.3) construction
  line L188 (-7, 0.75) -> (-7, 1.25)
  arc A28 (-7, 0.75) -> (-7, 1.25) centre (-7, 1) ccw
  line L189 (-6.6, 1.3) -> (-6.6, 0.7) construction
  arc A29 (-6.9, 0.7) -> (-6.9, 1.3) centre (-6.9, 1) ccw
  line L190 (-6.9, 1) -> (-6.9, 0.7) construction
  line L191 (-7, 0.7) -> (-7, 0.75)
  line L192 (-6.9, 0.7) -> (-7, 0.7)
  line L193 (-6.6, 0.7) -> (-7, 0.7) construction
  line L194 (-7, 0.7) -> (-6, 0.7)
  line L195 (-6, 0.7) -> (-6, 1.3)
  line L196 (-6, 1.3) -> (-7, 1.3)
  line L197 (-7, 1.3) -> (-7, 0.7)
  line L198 (-7, 0.25) -> (-7, 0.3)
  line L199 (-6.9, 0) -> (-6.9, 0.3) construction
  line L200 (-7, 0.3) -> (-6.9, 0.3)
  line L201 (-7, 0.3) -> (-6.6, 0.3) construction
  line L202 (-7, -0.25) -> (-7, 0.25)
  arc A30 (-7, -0.25) -> (-7, 0.25) centre (-7, 0) ccw
  line L203 (-6.6, 0.3) -> (-6.6, -0.3) construction
  arc A31 (-6.9, -0.3) -> (-6.9, 0.3) centre (-6.9, 0) ccw
  line L204 (-6.9, 0) -> (-6.9, -0.3) construction
  line L205 (-7, -0.3) -> (-7, -0.25)
  line L206 (-6.9, -0.3) -> (-7, -0.3)
  line L207 (-6.6, -0.3) -> (-7, -0.3) construction
  line L208 (-7, -0.3) -> (-6, -0.3)
  line L209 (-6, -0.3) -> (-6, 0.3)
  line L210 (-6, 0.3) -> (-7, 0.3)
  line L211 (-7, 0.3) -> (-7, -0.3)
  line L212 (-7, -0.75) -> (-7, -0.7)
  line L213 (-6.9, -1) -> (-6.9, -0.7) construction
  line L214 (-7, -0.7) -> (-6.9, -0.7)
  line L215 (-7, -0.7) -> (-6.6, -0.7) construction
  line L216 (-7, -1.25) -> (-7, -0.75)
  arc A32 (-7, -1.25) -> (-7, -0.75) centre (-7, -1) ccw
  line L217 (-6.6, -0.7) -> (-6.6, -1.3) construction
  arc A33 (-6.9, -1.3) -> (-6.9, -0.7) centre (-6.9, -1) ccw
  line L218 (-6.9, -1) -> (-6.9, -1.3) construction
  line L219 (-7, -1.3) -> (-7, -1.25)
  line L220 (-6.9, -1.3) -> (-7, -1.3)
  line L221 (-6.6, -1.3) -> (-7, -1.3) construction
  line L222 (-7, -1.3) -> (-6, -1.3)
  line L223 (-6, -1.3) -> (-6, -0.7)
  line L224 (-6, -0.7) -> (-7, -0.7)
  line L225 (-7, -0.7) -> (-7, -1.3)
  line L226 (-7, -1.75) -> (-7, -1.7)
  line L227 (-6.9, -2) -> (-6.9, -1.7) construction
  line L228 (-7, -1.7) -> (-6.9, -1.7)
  line L229 (-7, -1.7) -> (-6.6, -1.7) construction
  line L230 (-7, -2.25) -> (-7, -1.75)
  arc A34 (-7, -2.25) -> (-7, -1.75) centre (-7, -2) ccw
  line L231 (-6.6, -1.7) -> (-6.6, -2.3) construction
  arc A35 (-6.9, -2.3) -> (-6.9, -1.7) centre (-6.9, -2) ccw
  line L232 (-6.9, -2) -> (-6.9, -2.3) construction
  line L233 (-7, -2.3) -> (-7, -2.25)
  line L234 (-6.9, -2.3) -> (-7, -2.3)
  line L235 (-6.6, -2.3) -> (-7, -2.3) construction
  line L236 (-7, -2.3) -> (-6, -2.3)
  line L237 (-6, -2.3) -> (-6, -1.7)
  line L238 (-6, -1.7) -> (-7, -1.7)
  line L239 (-7, -1.7) -> (-7, -2.3)
  arc A36 (5.05, -4.8) -> (4.55, -4.8) centre (4.8, -4.8) ccw
  line L240 (5.05, -4.8) -> (5.1, -4.8)
  line L241 (5.1, -4.8) -> (5.1, -4.4) construction
  line L242 (5.1, -4.4) -> (4.5, -4.4) construction
  line L243 (4.5, -4.4) -> (4.5, -4.8) construction
  line L244 (4.5, -4.8) -> (4.55, -4.8)
  arc A37 (5.1, -4.7) -> (4.5, -4.7) centre (4.8, -4.7) ccw
  line L245 (4.8, -4.7) -> (5.1, -4.7) construction
  line L246 (4.8, -4.7) -> (4.5, -4.7) construction
  line L247 (4.5, -4.7) -> (4.5, -4.8)
  line L248 (5.1, -4.8) -> (5.1, -4.7)
  arc A38 (6.2, -4.8) -> (5.7, -4.8) centre (5.95, -4.8) ccw
  arc A39 (6.4, -4.8) -> (5.5, -4.8) centre (5.95, -4.8) ccw
  line L249 (5.5, -4.8) -> (5.7, -4.8)
  line L250 (6.2, -4.8) -> (6.4, -4.8)
  line L251 (4.55, -4.8) -> (5.05, -4.8)
  line L252 (5.7, -4.8) -> (6.2, -4.8)
  line L253 (4.5, -4.8) -> (4.5, -3.8)
  line L254 (4.5, -3.8) -> (5.1, -3.8)
  line L255 (5.1, -3.8) -> (5.1, -4.8)
  line L256 (3.5, -4.4) -> (3.5, -4.8) construction
  line L257 (3.5, -4.8) -> (3.5, -3.8)
  line L258 (3.5, -4.8) -> (3.55, -4.8)
  line L259 (3.8, -4.7) -> (3.5, -4.7) construction
  line L260 (4.05, -4.8) -> (4.1, -4.8)
  line L261 (3.8, -4.7) -> (4.1, -4.7) construction
  arc A40 (4.1, -4.7) -> (3.5, -4.7) centre (3.8, -4.7) ccw
  line L262 (3.5, -3.8) -> (4.1, -3.8)
  line L263 (4.1, -4.4) -> (3.5, -4.4) construction
  line L264 (4.1, -4.8) -> (4.1, -4.7)
  line L265 (4.1, -4.8) -> (4.1, -4.4) construction
  line L266 (4.1, -3.8) -> (4.1, -4.8)
  arc A41 (4.05, -4.8) -> (3.55, -4.8) centre (3.8, -4.8) ccw
  line L267 (3.5, -4.7) -> (3.5, -4.8)
  line L268 (3.55, -4.8) -> (4.05, -4.8)
  line L269 (2.5, -4.4) -> (2.5, -4.8) construction
  line L270 (2.5, -4.8) -> (2.5, -3.8)
  line L271 (2.5, -4.8) -> (2.55, -4.8)
  line L272 (2.8, -4.7) -> (2.5, -4.7) construction
  line L273 (3.05, -4.8) -> (3.1, -4.8)
  line L274 (2.8, -4.7) -> (3.1, -4.7) construction
  arc A42 (3.1, -4.7) -> (2.5, -4.7) centre (2.8, -4.7) ccw
  line L275 (2.5, -3.8) -> (3.1, -3.8)
  line L276 (3.1, -4.4) -> (2.5, -4.4) construction
  line L277 (3.1, -4.8) -> (3.1, -4.7)
  line L278 (3.1, -4.8) -> (3.1, -4.4) construction
  line L279 (3.1, -3.8) -> (3.1, -4.8)
  arc A43 (3.05, -4.8) -> (2.55, -4.8) centre (2.8, -4.8) ccw
  line L280 (2.5, -4.7) -> (2.5, -4.8)
  line L281 (2.55, -4.8) -> (3.05, -4.8)
  line L282 (1.5, -4.4) -> (1.5, -4.8) construction
  line L283 (1.5, -4.8) -> (1.5, -3.8)
  line L284 (1.5, -4.8) -> (1.55, -4.8)
  line L285 (1.8, -4.7) -> (1.5, -4.7) construction
  line L286 (2.05, -4.8) -> (2.1, -4.8)
  line L287 (1.8, -4.7) -> (2.1, -4.7) construction
  arc A44 (2.1, -4.7) -> (1.5, -4.7) centre (1.8, -4.7) ccw
  line L288 (1.5, -3.8) -> (2.1, -3.8)
  line L289 (2.1, -4.4) -> (1.5, -4.4) construction
  line L290 (2.1, -4.8) -> (2.1, -4.7)
  line L291 (2.1, -4.8) -> (2.1, -4.4) construction
  line L292 (2.1, -3.8) -> (2.1, -4.8)
  arc A45 (2.05, -4.8) -> (1.55, -4.8) centre (1.8, -4.8) ccw
  line L293 (1.5, -4.7) -> (1.5, -4.8)
  line L294 (1.55, -4.8) -> (2.05, -4.8)
  line L295 (0.5, -4.4) -> (0.5, -4.8) construction
  line L296 (0.5, -4.8) -> (0.5, -3.8)
  line L297 (0.5, -4.8) -> (0.55, -4.8)
  line L298 (0.8, -4.7) -> (0.5, -4.7) construction
  line L299 (1.05, -4.8) -> (1.1, -4.8)
  line L300 (0.8, -4.7) -> (1.1, -4.7) construction
  arc A46 (1.1, -4.7) -> (0.5, -4.7) centre (0.8, -4.7) ccw
  line L301 (0.5, -3.8) -> (1.1, -3.8)
  line L302 (1.1, -4.4) -> (0.5, -4.4) construction
  line L303 (1.1, -4.8) -> (1.1, -4.7)
  line L304 (1.1, -4.8) -> (1.1, -4.4) construction
  line L305 (1.1, -3.8) -> (1.1, -4.8)
  arc A47 (1.05, -4.8) -> (0.55, -4.8) centre (0.8, -4.8) ccw
  line L306 (0.5, -4.7) -> (0.5, -4.8)
  line L307 (0.55, -4.8) -> (1.05, -4.8)
  line L308 (-0.5, -4.4) -> (-0.5, -4.8) construction
  line L309 (-0.5, -4.8) -> (-0.5, -3.8)
  line L310 (-0.5, -4.8) -> (-0.45, -4.8)
  line L311 (-0.2, -4.7) -> (-0.5, -4.7) construction
  line L312 (0.05, -4.8) -> (0.1, -4.8)
  line L313 (-0.2, -4.7) -> (0.1, -4.7) construction
  arc A48 (0.1, -4.7) -> (-0.5, -4.7) centre (-0.2, -4.7) ccw
  line L314 (-0.5, -3.8) -> (0.1, -3.8)
  line L315 (0.1, -4.4) -> (-0.5, -4.4) construction
  line L316 (0.1, -4.8) -> (0.1, -4.7)
  line L317 (0.1, -4.8) -> (0.1, -4.4) construction
  line L318 (0.1, -3.8) -> (0.1, -4.8)
  arc A49 (0.05, -4.8) -> (-0.45, -4.8) centre (-0.2, -4.8) ccw
  line L319 (-0.5, -4.7) -> (-0.5, -4.8)
  line L320 (-0.45, -4.8) -> (0.05, -4.8)
  line L321 (-1.5, -4.4) -> (-1.5, -4.8) construction
  line L322 (-1.5, -4.8) -> (-1.5, -3.8)
  line L323 (-1.5, -4.8) -> (-1.45, -4.8)
  line L324 (-1.2, -4.7) -> (-1.5, -4.7) construction
  line L325 (-0.95, -4.8) -> (-0.9, -4.8)
  line L326 (-1.2, -4.7) -> (-0.9, -4.7) construction
  arc A50 (-0.9, -4.7) -> (-1.5, -4.7) centre (-1.2, -4.7) ccw
  line L327 (-1.5, -3.8) -> (-0.9, -3.8)
  line L328 (-0.9, -4.4) -> (-1.5, -4.4) construction
  line L329 (-0.9, -4.8) -> (-0.9, -4.7)
  line L330 (-0.9, -4.8) -> (-0.9, -4.4) construction
  line L331 (-0.9, -3.8) -> (-0.9, -4.8)
  arc A51 (-0.95, -4.8) -> (-1.45, -4.8) centre (-1.2, -4.8) ccw
  line L332 (-1.5, -4.7) -> (-1.5, -4.8)
  line L333 (-1.45, -4.8) -> (-0.95, -4.8)
  line L334 (-2.5, -4.4) -> (-2.5, -4.8) construction
  line L335 (-2.5, -4.8) -> (-2.5, -3.8)
  line L336 (-2.5, -4.8) -> (-2.45, -4.8)
  line L337 (-2.2, -4.7) -> (-2.5, -4.7) construction
  line L338 (-1.95, -4.8) -> (-1.9, -4.8)
  line L339 (-2.2, -4.7) -> (-1.9, -4.7) construction
  arc A52 (-1.9, -4.7) -> (-2.5, -4.7) centre (-2.2, -4.7) ccw
  line L340 (-2.5, -3.8) -> (-1.9, -3.8)
  line L341 (-1.9, -4.4) -> (-2.5, -4.4) construction
  line L342 (-1.9, -4.8) -> (-1.9, -4.7)
  line L343 (-1.9, -4.8) -> (-1.9, -4.4) construction
  line L344 (-1.9, -3.8) -> (-1.9, -4.8)
  arc A53 (-1.95, -4.8) -> (-2.45, -4.8) centre (-2.2, -4.8) ccw
  line L345 (-2.5, -4.7) -> (-2.5, -4.8)
  line L346 (-2.45, -4.8) -> (-1.95, -4.8)
  line L347 (-3.5, -4.4) -> (-3.5, -4.8) construction
  line L348 (-3.5, -4.8) -> (-3.5, -3.8)
  line L349 (-3.5, -4.8) -> (-3.45, -4.8)
  line L350 (-3.2, -4.7) -> (-3.5, -4.7) construction
  line L351 (-2.95, -4.8) -> (-2.9, -4.8)
  line L352 (-3.2, -4.7) -> (-2.9, -4.7) construction
  arc A54 (-2.9, -4.7) -> (-3.5, -4.7) centre (-3.2, -4.7) ccw
  line L353 (-3.5, -3.8) -> (-2.9, -3.8)
  line L354 (-2.9, -4.4) -> (-3.5, -4.4) construction
  line L355 (-2.9, -4.8) -> (-2.9, -4.7)
  line L356 (-2.9, -4.8) -> (-2.9, -4.4) construction
  line L357 (-2.9, -3.8) -> (-2.9, -4.8)
  arc A55 (-2.95, -4.8) -> (-3.45, -4.8) centre (-3.2, -4.8) ccw
  line L358 (-3.5, -4.7) -> (-3.5, -4.8)
  line L359 (-3.45, -4.8) -> (-2.95, -4.8)
  line L360 (-4.5, -4.4) -> (-4.5, -4.8) construction
  line L361 (-4.5, -4.8) -> (-4.5, -3.8)
  line L362 (-4.5, -4.8) -> (-4.45, -4.8)
  line L363 (-4.2, -4.7) -> (-4.5, -4.7) construction
  line L364 (-3.95, -4.8) -> (-3.9, -4.8)
  line L365 (-4.2, -4.7) -> (-3.9, -4.7) construction
  arc A56 (-3.9, -4.7) -> (-4.5, -4.7) centre (-4.2, -4.7) ccw
  line L366 (-4.5, -3.8) -> (-3.9, -3.8)
  line L367 (-3.9, -4.4) -> (-4.5, -4.4) construction
  line L368 (-3.9, -4.8) -> (-3.9, -4.7)
  line L369 (-3.9, -4.8) -> (-3.9, -4.4) construction
  line L370 (-3.9, -3.8) -> (-3.9, -4.8)
  arc A57 (-3.95, -4.8) -> (-4.45, -4.8) centre (-4.2, -4.8) ccw
  line L371 (-4.5, -4.7) -> (-4.5, -4.8)
  line L372 (-4.45, -4.8) -> (-3.95, -4.8)
  line L373 (-5.5, -4.4) -> (-5.5, -4.8) construction
  line L374 (-5.5, -4.8) -> (-5.5, -3.8)
  line L375 (-5.5, -4.8) -> (-5.45, -4.8)
  line L376 (-5.2, -4.7) -> (-5.5, -4.7) construction
  line L377 (-4.95, -4.8) -> (-4.9, -4.8)
  line L378 (-5.2, -4.7) -> (-4.9, -4.7) construction
  arc A58 (-4.9, -4.7) -> (-5.5, -4.7) centre (-5.2, -4.7) ccw
  line L379 (-5.5, -3.8) -> (-4.9, -3.8)
  line L380 (-4.9, -4.4) -> (-5.5, -4.4) construction
  line L381 (-4.9, -4.8) -> (-4.9, -4.7)
  line L382 (-4.9, -4.8) -> (-4.9, -4.4) construction
  line L383 (-4.9, -3.8) -> (-4.9, -4.8)
  arc A59 (-4.95, -4.8) -> (-5.45, -4.8) centre (-5.2, -4.8) ccw
  line L384 (-5.5, -4.7) -> (-5.5, -4.8)
  line L385 (-5.45, -4.8) -> (-4.95, -4.8)
  line L386 (-6.5, -4.4) -> (-6.5, -4.8) construction
  line L387 (-6.5, -4.8) -> (-6.5, -3.8)
  line L388 (-6.5, -4.8) -> (-6.45, -4.8)
  line L389 (-6.2, -4.7) -> (-6.5, -4.7) construction
  line L390 (-5.95, -4.8) -> (-5.9, -4.8)
  line L391 (-6.2, -4.7) -> (-5.9, -4.7) construction
  arc A60 (-5.9, -4.7) -> (-6.5, -4.7) centre (-6.2, -4.7) ccw
  line L392 (-6.5, -3.8) -> (-5.9, -3.8)
  line L393 (-5.9, -4.4) -> (-6.5, -4.4) construction
  line L394 (-5.9, -4.8) -> (-5.9, -4.7)
  line L395 (-5.9, -4.8) -> (-5.9, -4.4) construction
  line L396 (-5.9, -3.8) -> (-5.9, -4.8)
  arc A61 (-5.95, -4.8) -> (-6.45, -4.8) centre (-6.2, -4.8) ccw
  line L397 (-6.5, -4.7) -> (-6.5, -4.8)
  line L398 (-6.45, -4.8) -> (-5.95, -4.8)
  line L399 (5.5, -4.8) -> (6.4, -4.8)
  line L400 (6.4, -4.8) -> (6.4, -3.8)
  line L401 (6.4, -3.8) -> (5.5, -3.8)
  line L402 (5.5, -3.8) -> (5.5, -4.8)
  point P0 (4.8, 4.4)
  point P1 (-6.6, 2)
  point P2 (3.8, 4.4)
  point P3 (2.8, 4.4)
  point P4 (1.8, 4.4)
  point P5 (0.8, 4.4)
  point P6 (-0.2, 4.4)
  point P7 (-1.2, 4.4)
  point P8 (-2.2, 4.4)
  point P9 (-3.2, 4.4)
  point P10 (-4.2, 4.4)
  point P11 (-5.2, 4.4)
  point P12 (-6.2, 4.4)
  point P13 (-6.6, 1)
  point P14 (-6.6, 0)
  point P15 (-6.6, -1)
  point P16 (-6.6, -2)
  point P17 (4.8, -4.4)
  point P18 (3.8, -4.4)
  point P19 (2.8, -4.4)
  point P20 (1.8, -4.4)
  point P21 (0.8, -4.4)
  point P22 (-0.2, -4.4)
  point P23 (-1.2, -4.4)
  point P24 (-2.2, -4.4)
  point P25 (-3.2, -4.4)
  point P26 (-4.2, -4.4)
  point P27 (-5.2, -4.4)
  point P28 (-6.2, -4.4)
  dimension "d1051" = 0.25
  dimension "d1052" = 0.6
  dimension "d1053" = 0.4
  dimension "d1054" = 0.25
  dimension "d1055" = 0.45
  dimension "d1056" = 1.15
  dimension "d1057" = 14
  dimension "d1058" = 9.6
  dimension "d1104" = 0.25
  dimension "d1105" = 0.6
  dimension "d1106" = 0.4
  dimension "d1107" = 2.8
  dimension "d1126" = 1
  dimension "d1135" = 1
  dimension "d1140" = 0.8
  dimension "d1141" = 1
  dimension "d1142" = 1
  dimension "d1145" = 1
  constraints: 806 end point, 164 symmetric about line, 126 point on circle, 89 point on line, 62 centre point, 14 perpendicular, 10 parallel, 9 horizontal alignment, 7 midpoint, 6 horizontal, 5 collinear, 3 coincident, 3 vertical alignment, 2 vertical, 456 other
  measures "d1051" radius of A0
  measures "d1052" distance between parallel lines of L1 L3
  measures "d1053" distance of L2.end L3.end
  measures "d1054" radius of A2
  measures "d1055" radius of A3
  measures "d1056" distance of A0.centre A2.centre
  measures "d1057" distance of L13.end L12.end
  measures "d1058" distance of L12.end L11.end
  measures "d1104" radius of A4
  measures "d1105" distance between parallel lines of L23 L29
  measures "d1106" distance of L25.end L27.start
  measures "d1107" distance of L13.end A4.centre
  measures "d1126" distance from line of A0.centre L31